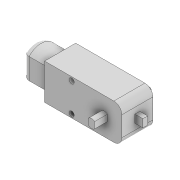
# Autodesk Inventor part: DC Hobby Motor
Saved by Autodesk Inventor 2022 (Build 260153000, 153)
## iProperties
Created: 2024-05-31
Part Number: DC Hobby Motor
Material: Generic
Document SubType Name: Modeling
Designer: david
Density: 1 g/cm^3
Appearance: Default
Author: david
Autodesk Inventor part; units mm, degrees
ref_plane "YZ Plane" through (0, 0, 0) normal (1, 0, 0) x (0, 1, 0)
ref_plane "XZ Plane" through (0, 0, 0) normal (0, 1, 0) x (-1, 0, 0)
ref_plane "XY Plane" through (0, 0, 0) normal (0, 0, 1) x (1, 0, 0)
sketch "Sketch1" plane through (0, 0, 0) normal (0, 1, 0) x (-1, 0, 0)
  line L0 (24.25, 9.75) -> (-24.25, 9.75)
  line L1 (-24.25, 9.75) -> (-24.25, -9.75)
  line L2 (-24.25, -9.75) -> (24.25, -9.75)
  line L3 (24.25, -9.75) -> (24.25, 9.75)
  line L4 (24.25, 9.75) -> (-24.25, -9.75) construction
  line L5 (-24.25, 9.75) -> (24.25, -9.75) construction
  point P0 (0, 0)
  dimension "d0" = 19.5
  dimension "d1" = 48.5
  constraints: 12 end point, 2 midpoint, 2 parallel, 1 horizontal, 1 perpendicular
  measures "d0" distance of L0.end L1.end
  measures "d1" distance of L1.end L2.end
extrude "Extrusion1" add sketch "Sketch1" along normal mid plane 22.5
sketch "Sketch2" plane through (24.25, -11.25, -9.75) normal (1, 0, 0) x (0, 0, -1)
  line L0 (-11.25, 8.75) -> (-8.25, 8.75)
  line L1 (-8.25, 8.75) -> (-8.25, 13.75)
  line L2 (-8.25, 13.75) -> (-11.25, 13.75)
  line L3 (-11.25, 13.75) -> (-11.25, 8.75)
  line L4 (-11.25, 8.75) -> (-8.25, 13.75) construction
  line L5 (-8.25, 8.75) -> (-11.25, 13.75) construction
  point P0 (-9.75, 11.25)
  dimension "d4" = 3
  dimension "d5" = 5
  constraints: 12 end point, 2 midpoint, 2 parallel, 1 horizontal, 1 perpendicular
  measures "d4" distance of L1.end L2.end
  measures "d5" distance of L0.end L1.end
extrude "Extrusion2" add sketch "Sketch2" along normal blind 5
fillet "Fillet1" radius 5 2 edges at (24.25, 11.25, 0) (24.25, -11.25, 0)
sketch "Sketch3" plane through (-24.25, -11.25, 9.75) normal (-1, 0, 0) x (0, 0, 1)
  arc A0 (-2.25, 17.8644) -> (-17.25, 17.8644) centre (-9.75, 11.25) ccw
  line L0 (-2.25, 17.8644) -> (-17.25, 17.8644) construction
  line L1 (-17.25, 17.8644) -> (-17.25, 4.6356)
  line L2 (-17.25, 4.6356) -> (-2.25, 4.6356) construction
  line L3 (-2.25, 4.6356) -> (-2.25, 17.8644)
  line L4 (-2.25, 17.8644) -> (-17.25, 4.6356) construction
  line L5 (-17.25, 17.8644) -> (-2.25, 4.6356) construction
  arc A1 (-2.25, 4.6356) -> (-2.25, 17.8644) centre (-9.75, 11.25) ccw construction
  arc A2 (-17.25, 4.6356) -> (-2.25, 4.6356) centre (-9.75, 11.25) ccw
  arc A3 (-17.25, 17.8644) -> (-17.25, 4.6356) centre (-9.75, 11.25) ccw construction
  dimension "d9" = 20
  dimension "d10" = 15
  constraints: 12 end point, 8 point on circle, 4 centre point, 2 midpoint, 2 parallel, 1 coincident, 1 horizontal, 1 perpendicular
  measures "d9" diameter of A0
  measures "d10" distance of L1.end L2.end
extrude "Extrusion3" add sketch "Sketch3" along normal blind 16
fillet "Fillet2" radius 4 4 edges at (-40.25, -10, 0) (-40.25, 0, 7.5) (-40.25, 0, -7.5) (-40.25, 10, 0)
sketch "Sketch4" plane through (-24.25, -11.25, -9.75) normal (0, 0, -1) x (-1, 0, 0)
  arc A0 (-39.3875, 13.25) -> (-39.3875, 9.25) centre (-37.5, 11.25) ccw construction
  line L0 (-39.3875, 9.25) -> (-35.6125, 9.25) construction
  line L1 (-35.6125, 9.25) -> (-35.6125, 13.25)
  line L2 (-35.6125, 13.25) -> (-39.3875, 13.25) construction
  line L3 (-39.3875, 13.25) -> (-39.3875, 9.25)
  line L4 (-39.3875, 9.25) -> (-35.6125, 13.25) construction
  line L5 (-35.6125, 9.25) -> (-37.5, 11.25) construction
  arc A1 (-35.6125, 13.25) -> (-39.3875, 13.25) centre (-37.5, 11.25) ccw
  arc A2 (-35.6125, 9.25) -> (-35.6125, 13.25) centre (-37.5, 11.25) ccw construction
  arc A3 (-39.3875, 9.25) -> (-35.6125, 9.25) centre (-37.5, 11.25) ccw
  line L6 (-37.5, 11.25) -> (-39.3875, 13.25) construction
  line L7 (0, 0) -> (-43.5, 0) projected
  line L8 (-48.5, 5) -> (-48.5, 17.5) projected
  point P0 (-24.25, 11.25)
  dimension "d14" = 5.5
  dimension "d15" = 4
  dimension "d16" = 11.25
  dimension "d17" = 11
  constraints: 14 end point, 8 point on circle, 4 centre point, 2 parallel, 1 coincident, 1 horizontal, 1 midpoint, 1 perpendicular
  measures "d14" diameter of A0
  measures "d15" distance of L1.end L0.end
  measures "d16" distance from line of L7 point (-37.5, 11.25)
  measures "d17" distance from line of point (-37.5, 11.25) L8
extrude "Extrusion4" add sketch "Sketch4" along normal blind 8
mirror "Mirror1" about plane through (0, 0, 0) normal (0, 0, 1) of "Extrusion4"
sketch "Sketch5" plane through (-24.25, -11.25, -9.75) normal (0, 0, -1) x (-1, 0, 0)
  line L0 (0, 0) -> (-43.5, 0) projected
  line L1 (-35.6125, 13.25) -> (-35.6125, 9.25) projected
  arc A0 (-39.3875, 9.25) -> (-35.6125, 9.25) centre (-37.5, 11.25) ccw projected
  line L2 (-39.3875, 9.25) -> (-39.3875, 13.25) projected
  arc A1 (-35.6125, 13.25) -> (-39.3875, 13.25) centre (-37.5, 11.25) ccw projected
  arc A2 (-48.5, 5) -> (-43.5, 0) centre (-43.5, 5) ccw projected
  line L3 (-48.5, 5) -> (-48.5, 17.5) projected
  arc A3 (-43.5, 22.5) -> (-48.5, 17.5) centre (-43.5, 17.5) ccw projected
  line L4 (-43.5, 22.5) -> (0, 22.5) projected
  line L5 (0, 22.5) -> (0, 0) projected
  line L6 (0, 0) -> (-43.5, 0) projected
  line L7 (0, 0) -> (0, 22.5) projected
  line L8 (0, 11.25) -> (-48.5, 11.25) construction
  line L9 (-48.5, 13.75) -> (-48.5, 8.75) projected
  point P0 (-24.25, 11.25)
  point P1 (-17, 2.25)
  point P2 (-17, 20.25)
  dimension "d21" = 18
  dimension "d22" = 17
  constraints: 2 end point, 2 midpoint, 1 symmetric about line, 1 vertical alignment
  measures "d21" distance of point (-17, 2.25) point (-17, 20.25)
  measures "d22" distance from line of L5 point (-17, 20.25)
hole "Hole1" at (-7.25, -9, -9.75) at (-7.25, 9, -9.75) direction (0, 0, 1) diameter 3.2 end through all
body "Solid1"
